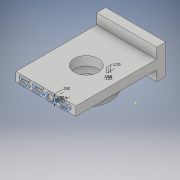
# Autodesk Inventor part: RSL mount
Saved by Autodesk Inventor 2019 (Build 230136000, 136)
## iProperties
Created: 2019-02-11
Part Number: RSL mount
Material: Generic
Document SubType Name: Modeling
Designer: josh
Density: 1 g/cm^3
Appearance: Default
Author: josh
Autodesk Inventor part; units mm, degrees
sketch "Sketch1" plane through (0, 0, 0) normal (0, 0, 1) x (1, 0, 0)
  line L0 (50.8, 31.75) -> (50.8, 57.15)
  line L1 (0, 57.15) -> (0, 31.75)
  line L2 (0, 57.15) -> (0, 48.26)
  line L3 (0, 31.75) -> (0, 40.64)
  line L4 (0, 40.64) -> (50.8, 40.64)
  line L5 (50.8, 48.26) -> (0, 48.26)
  line L6 (0, 40.64) -> (0, 31.75)
  line L7 (0, 31.75) -> (50.8, 31.75)
  line L8 (0, 48.26) -> (0, 57.15)
  line L9 (0, 57.15) -> (50.8, 57.15)
  point P0 (0, 0)
  dimension "d30" = 7.62
  dimension "d33" = 8.89
  dimension "d34" = 8.89
  constraints: 20 end point, 4 perpendicular, 4 point on line, 1 parallel
  measures "d30" distance between parallel lines of L4 L5
  measures "d33" distance of L1.end L3.end
  measures "d34" distance of L1.start L2.end
sketch "Sketch1 outline for Extrusion1" plane through (0, 0, 0) normal (0, 0, 1) x (1, 0, 0)
  line L0 (50.8, 57.15) -> (0, 57.15)
  line L1 (0, 57.15) -> (0, 31.75)
  line L2 (0, 31.75) -> (50.8, 31.75)
  line L3 (50.8, 31.75) -> (50.8, 57.15)
extrude "Extrusion1" add sketch "Sketch1 outline for Extrusion1" along normal blind 7.62
sketch "Sketch1 outline for Extrusion2" plane through (0, 0, 0) normal (0, 0, 1) x (1, 0, 0)
  line L0 (50.8, 48.26) -> (0, 48.26)
  line L1 (50.8, 40.64) -> (50.8, 48.26)
  line L2 (0, 40.64) -> (50.8, 40.64)
  line L3 (0, 48.26) -> (0, 40.64)
extrude "Extrusion2" add sketch "Sketch1 outline for Extrusion2" along normal blind 76.2
sketch "Sketch3" plane through (0, 48.26, 7.62) normal (0, 1, 0) x (1, 0, 0)
  line L0 (0, 0) -> (0, -68.58) projected
  line L1 (0, -34.29) -> (50.8, -34.29)
  line L2 (50.8, 0) -> (50.8, -68.58) projected
  circle A0 centre (25.4, -34.29) radius 10.16
  point P0 (0, 7.62)
  dimension "d8" = 20.32
  constraints: 3 midpoint, 2 end point, 1 centre point
  measures "d8" diameter of A0
sketch "Sketch3 outline for Extrusion3" plane through (0, 48.26, 7.62) normal (0, 1, 0) x (1, 0, 0)
  circle A0 centre (25.4, -34.29) radius 10.16
extrude "Extrusion3" cut sketch "Sketch3 outline for Extrusion3" against normal blind 50.8
sketch "Sketch4" plane through (0, 0, 76.2) normal (0, 0, 1) x (1, 0, 0)
  line L0 (2.114668, 47.727642) -> (47.879129, 47.727642) construction
  line L1 (47.879129, 47.727642) -> (47.879129, 41.3797) construction
  line L2 (47.879129, 41.3797) -> (2.114668, 41.3797) construction
  line L3 (2.114668, 41.3797) -> (2.114668, 47.727642) construction
  spline S0 degree 2 poles (12.464037, 43.444634) (12.464037, 43.004971) (11.757612, 42.254086) (11.125288, 41.977444) knots 0 0 0 1 2 2 2
  spline S1 degree 2 poles (11.125288, 41.977444) (10.478143, 41.700803) (8.566351, 41.3797) (7.375803, 41.3797) knots 0 0 0 1 2 2 2
  spline S2 degree 2 poles (7.375803, 41.3797) (6.279116, 41.3797) (4.159842, 41.572362) (3.384257, 41.725503) knots 0 0 0 1 2 2 2
  line L4 (3.384257, 41.725503) -> (3.384257, 42.590008)
  line L5 (3.384257, 42.590008) -> (3.527518, 42.590008)
  spline S3 degree 2 poles (3.527518, 42.590008) (3.764639, 42.520848) (4.643965, 42.343007) (5.177489, 42.263966) knots 0 0 0 1 2 2 2
  spline S4 degree 2 poles (5.177489, 42.263966) (5.780173, 42.179986) (6.782999, 42.086125) (7.405443, 42.086125) knots 0 0 0 1 2 2 2
  spline S5 degree 2 poles (7.405443, 42.086125) (8.018007, 42.086125) (9.188795, 42.263966) (9.608698, 42.456628) knots 0 0 0 1 2 2 2
  spline S6 degree 2 poles (9.608698, 42.456628) (9.98414, 42.639409) (10.384283, 43.123532) (10.384283, 43.449574) knots 0 0 0 1 2 2 2
  spline S7 degree 2 poles (10.384283, 43.449574) (10.384283, 43.775616) (9.94462, 44.190579) (9.524717, 44.3289) knots 0 0 0 1 2 2 2
  spline S8 degree 2 poles (9.524717, 44.3289) (9.085054, 44.482041) (7.805586, 44.610482) (7.015181, 44.610482) knots 0 0 0 1 2 2 2
  spline S9 degree 2 poles (7.015181, 44.610482) (6.185255, 44.610482) (4.510584, 44.506741) (4.006701, 44.462281) knots 0 0 0 1 2 2 2
  line L6 (4.006701, 44.462281) -> (4.006701, 47.604141)
  line L7 (4.006701, 47.604141) -> (12.370176, 47.604141)
  line L8 (12.370176, 47.604141) -> (12.370176, 46.887837)
  line L9 (12.370176, 46.887837) -> (5.982714, 46.887837)
  line L10 (5.982714, 46.887837) -> (5.982714, 45.262566)
  spline S10 degree 2 poles (5.982714, 45.262566) (6.353216, 45.282326) (7.069521, 45.297146) (7.365923, 45.297146) knots 0 0 0 1 2 2 2
  spline S11 degree 2 poles (7.365923, 45.297146) (8.531771, 45.297146) (10.152101, 45.144005) (10.898046, 44.916764) knots 0 0 0 1 2 2 2
  spline S12 degree 2 poles (10.898046, 44.916764) (11.653871, 44.689522) (12.464037, 43.997918) (12.464037, 43.444634) knots 0 0 0 1 2 2 2
  spline S13 degree 2 poles (23.905152, 43.444634) (23.905152, 43.004971) (23.198727, 42.254086) (22.566403, 41.977444) knots 0 0 0 1 2 2 2
  spline S14 degree 2 poles (22.566403, 41.977444) (21.919259, 41.700803) (20.007466, 41.3797) (18.816918, 41.3797) knots 0 0 0 1 2 2 2
  spline S15 degree 2 poles (18.816918, 41.3797) (17.720231, 41.3797) (15.600957, 41.572362) (14.825372, 41.725503) knots 0 0 0 1 2 2 2
  line L11 (14.825372, 41.725503) -> (14.825372, 42.590008)
  line L12 (14.825372, 42.590008) -> (14.968633, 42.590008)
  spline S16 degree 2 poles (14.968633, 42.590008) (15.205755, 42.520848) (16.08508, 42.343007) (16.618604, 42.263966) knots 0 0 0 1 2 2 2
  spline S17 degree 2 poles (16.618604, 42.263966) (17.221288, 42.179986) (18.224114, 42.086125) (18.846558, 42.086125) knots 0 0 0 1 2 2 2
  spline S18 degree 2 poles (18.846558, 42.086125) (19.459123, 42.086125) (20.62991, 42.263966) (21.049813, 42.456628) knots 0 0 0 1 2 2 2
  spline S19 degree 2 poles (21.049813, 42.456628) (21.425255, 42.639409) (21.825398, 43.123532) (21.825398, 43.449574) knots 0 0 0 1 2 2 2
  spline S20 degree 2 poles (21.825398, 43.449574) (21.825398, 43.775616) (21.385735, 44.190579) (20.965832, 44.3289) knots 0 0 0 1 2 2 2
  spline S21 degree 2 poles (20.965832, 44.3289) (20.52617, 44.482041) (19.246701, 44.610482) (18.456296, 44.610482) knots 0 0 0 1 2 2 2
  spline S22 degree 2 poles (18.456296, 44.610482) (17.62637, 44.610482) (15.951699, 44.506741) (15.447816, 44.462281) knots 0 0 0 1 2 2 2
  line L13 (15.447816, 44.462281) -> (15.447816, 47.604141)
  line L14 (15.447816, 47.604141) -> (23.811291, 47.604141)
  line L15 (23.811291, 47.604141) -> (23.811291, 46.887837)
  line L16 (23.811291, 46.887837) -> (17.423829, 46.887837)
  line L17 (17.423829, 46.887837) -> (17.423829, 45.262566)
  spline S23 degree 2 poles (17.423829, 45.262566) (17.794332, 45.282326) (18.510636, 45.297146) (18.807038, 45.297146) knots 0 0 0 1 2 2 2
  spline S24 degree 2 poles (18.807038, 45.297146) (19.972886, 45.297146) (21.593217, 45.144005) (22.339161, 44.916764) knots 0 0 0 1 2 2 2
  spline S25 degree 2 poles (22.339161, 44.916764) (23.094986, 44.689522) (23.905152, 43.997918) (23.905152, 43.444634) knots 0 0 0 1 2 2 2
  spline S26 degree 2 poles (35.588329, 44.556141) (35.588329, 42.916051) (33.202293, 41.3797) (30.717457, 41.3797) knots 0 0 0 1 2 2 2
  spline S27 degree 2 poles (30.717457, 41.3797) (28.19804, 41.3797) (25.846585, 42.945691) (25.846585, 44.551201) knots 0 0 0 1 2 2 2
  spline S28 degree 2 poles (25.846585, 44.551201) (25.846585, 46.201172) (28.23262, 47.727642) (30.717457, 47.727642) knots 0 0 0 1 2 2 2
  spline S29 degree 2 poles (30.717457, 47.727642) (33.236873, 47.727642) (35.588329, 46.146832) (35.588329, 44.556141) knots 0 0 0 1 2 2 2
  spline S30 degree 2 poles (32.965171, 42.698689) (33.261573, 43.000031) (33.508575, 43.928757) (33.508575, 44.556141) knots 0 0 0 1 2 2 2
  spline S31 degree 2 poles (33.508575, 44.556141) (33.508575, 45.183525) (33.261573, 46.107312) (32.955291, 46.418534) knots 0 0 0 1 2 2 2
  spline S32 degree 2 poles (32.955291, 46.418534) (32.649009, 46.729756) (31.577022, 47.050858) (30.717457, 47.050858) knots 0 0 0 1 2 2 2
  spline S33 degree 2 poles (30.717457, 47.050858) (29.867771, 47.050858) (28.776024, 46.729756) (28.459862, 46.408654) knots 0 0 0 1 2 2 2
  spline S34 degree 2 poles (28.459862, 46.408654) (28.15358, 46.097431) (27.926338, 45.148945) (27.926338, 44.551201) knots 0 0 0 1 2 2 2
  spline S35 degree 2 poles (27.926338, 44.551201) (27.926338, 43.908997) (28.118999, 43.049431) (28.449982, 42.713509) knots 0 0 0 1 2 2 2
  spline S36 degree 2 poles (28.449982, 42.713509) (28.746384, 42.397347) (29.838131, 42.056485) (30.717457, 42.056485) knots 0 0 0 1 2 2 2
  spline S37 degree 2 poles (30.717457, 42.056485) (31.567142, 42.056485) (32.658889, 42.377587) (32.965171, 42.698689) knots 0 0 0 1 2 2 2
  spline S38 degree 2 poles (37.124679, 45.623188) (37.124679, 46.092491) (37.890384, 46.873017) (38.557288, 47.154598) knots 0 0 0 1 2 2 2
  spline S39 degree 2 poles (38.557288, 47.154598) (39.189612, 47.4263) (41.022364, 47.727642) (41.96591, 47.727642) knots 0 0 0 1 2 2 2
  spline S40 degree 2 poles (41.96591, 47.727642) (43.018137, 47.727642) (44.727389, 47.44606) (45.349833, 47.179299) knots 0 0 0 1 2 2 2
  spline S41 degree 2 poles (45.349833, 47.179299) (46.140238, 46.843376) (47.009684, 45.756569) (47.009684, 44.921704) knots 0 0 0 1 2 2 2
  spline S42 degree 2 poles (47.009684, 44.921704) (47.009684, 44.165879) (46.159998, 42.81231) (45.330073, 42.362767) knots 0 0 0 1 2 2 2
  spline S43 degree 2 poles (45.330073, 42.362767) (44.450747, 41.888524) (41.985671, 41.389581) (40.172679, 41.389581) knots 0 0 0 1 2 2 2
  spline S44 degree 2 poles (40.172679, 41.389581) (39.762656, 41.389581) (38.84381, 41.424161) (38.443667, 41.473561) knots 0 0 0 1 2 2 2
  line L18 (38.443667, 41.473561) -> (38.443667, 42.259026)
  line L19 (38.443667, 42.259026) -> (38.547408, 42.259026)
  spline S45 degree 2 poles (38.547408, 42.259026) (38.80429, 42.199746) (39.886157, 42.096005) (40.449321, 42.096005) knots 0 0 0 1 2 2 2
  spline S46 degree 2 poles (40.449321, 42.096005) (42.454974, 42.096005) (44.752089, 43.153172) (44.90523, 44.131299) knots 0 0 0 1 2 2 2
  spline S47 degree 2 poles (44.90523, 44.131299) (44.085184, 43.908997) (42.598235, 43.706456) (41.728789, 43.706456) knots 0 0 0 1 2 2 2
  spline S48 degree 2 poles (41.728789, 43.706456) (40.879103, 43.706456) (39.490954, 43.854657) (38.78453, 44.067078) knots 0 0 0 1 2 2 2
  spline S49 degree 2 poles (38.78453, 44.067078) (37.964484, 44.31902) (37.124679, 45.084725) (37.124679, 45.623188) knots 0 0 0 1 2 2 2
  spline S50 degree 2 poles (44.95463, 45.104485) (44.95463, 45.721989) (44.381586, 46.502514) (43.882643, 46.714936) knots 0 0 0 1 2 2 2
  spline S51 degree 2 poles (43.882643, 46.714936) (43.42816, 46.912537) (42.509314, 47.060738) (41.95603, 47.060738) knots 0 0 0 1 2 2 2
  spline S52 degree 2 poles (41.95603, 47.060738) (40.696322, 47.060738) (39.204432, 46.339493) (39.204432, 45.657769) knots 0 0 0 1 2 2 2
  spline S53 degree 2 poles (39.204432, 45.657769) (39.204432, 45.272446) (39.693496, 44.773503) (40.246779, 44.595662) knots 0 0 0 1 2 2 2
  spline S54 degree 2 poles (40.246779, 44.595662) (40.637042, 44.467221) (41.620108, 44.38324) (42.183272, 44.38324) knots 0 0 0 1 2 2 2
  spline S55 degree 2 poles (42.183272, 44.38324) (42.835356, 44.38324) (44.351946, 44.566021) (44.91511, 44.719162) knots 0 0 0 1 2 2 2
  spline S56 degree 2 poles (44.91511, 44.719162) (44.92499, 44.778443) (44.95463, 44.980984) (44.95463, 45.104485) knots 0 0 0 1 2 2 2
  point P0 (0, 0)
  constraints: 2 other
sketch "Sketch4 outline for Emboss1" plane through (0, 0, 76.2) normal (0, 0, 1) x (1, 0, 0)
  spline S0 degree 2 poles (12.464037, 43.444634) (12.464037, 43.004971) (11.757612, 42.254086) (11.125288, 41.977444) knots 0 0 0 0.5 1 1 1
  spline S1 degree 2 poles (11.125288, 41.977444) (10.478143, 41.700803) (8.566351, 41.3797) (7.375803, 41.3797) knots 0 0 0 0.5 1 1 1
  spline S2 degree 2 poles (7.375803, 41.3797) (6.279116, 41.3797) (4.159842, 41.572362) (3.384257, 41.725503) knots 0 0 0 0.5 1 1 1
  line L0 (3.384257, 41.725503) -> (3.384257, 42.590008)
  line L1 (3.384257, 42.590008) -> (3.527518, 42.590008)
  spline S3 degree 2 poles (3.527518, 42.590008) (3.764639, 42.520848) (4.643965, 42.343007) (5.177489, 42.263966) knots 0 0 0 0.5 1 1 1
  spline S4 degree 2 poles (5.177489, 42.263966) (5.780173, 42.179986) (6.782999, 42.086125) (7.405443, 42.086125) knots 0 0 0 0.5 1 1 1
  spline S5 degree 2 poles (7.405443, 42.086125) (8.018007, 42.086125) (9.188795, 42.263966) (9.608698, 42.456628) knots 0 0 0 0.5 1 1 1
  spline S6 degree 2 poles (9.608698, 42.456628) (9.98414, 42.639409) (10.384283, 43.123532) (10.384283, 43.449574) knots 0 0 0 0.5 1 1 1
  spline S7 degree 2 poles (10.384283, 43.449574) (10.384283, 43.775616) (9.94462, 44.190579) (9.524717, 44.3289) knots 0 0 0 0.5 1 1 1
  spline S8 degree 2 poles (9.524717, 44.3289) (9.085054, 44.482041) (7.805586, 44.610482) (7.015181, 44.610482) knots 0 0 0 0.5 1 1 1
  spline S9 degree 2 poles (7.015181, 44.610482) (6.185255, 44.610482) (4.510584, 44.506741) (4.006701, 44.462281) knots 0 0 0 0.5 1 1 1
  line L2 (4.006701, 44.462281) -> (4.006701, 47.604141)
  line L3 (4.006701, 47.604141) -> (12.370176, 47.604141)
  line L4 (12.370176, 47.604141) -> (12.370176, 46.887837)
  line L5 (12.370176, 46.887837) -> (5.982714, 46.887837)
  line L6 (5.982714, 46.887837) -> (5.982714, 45.262566)
  spline S10 degree 2 poles (5.982714, 45.262566) (6.353216, 45.282326) (7.069521, 45.297146) (7.365923, 45.297146) knots 0 0 0 0.5 1 1 1
  spline S11 degree 2 poles (7.365923, 45.297146) (8.531771, 45.297146) (10.152101, 45.144005) (10.898046, 44.916764) knots 0 0 0 0.5 1 1 1
  spline S12 degree 2 poles (10.898046, 44.916764) (11.653871, 44.689522) (12.464037, 43.997918) (12.464037, 43.444634) knots 0 0 0 0.5 1 1 1
  spline S13 degree 2 poles (23.905152, 43.444634) (23.905152, 43.004971) (23.198727, 42.254086) (22.566403, 41.977444) knots 0 0 0 0.5 1 1 1
  spline S14 degree 2 poles (22.566403, 41.977444) (21.919259, 41.700803) (20.007466, 41.3797) (18.816918, 41.3797) knots 0 0 0 0.5 1 1 1
  spline S15 degree 2 poles (18.816918, 41.3797) (17.720231, 41.3797) (15.600957, 41.572362) (14.825372, 41.725503) knots 0 0 0 0.5 1 1 1
  line L7 (14.825372, 41.725503) -> (14.825372, 42.590008)
  line L8 (14.825372, 42.590008) -> (14.968633, 42.590008)
  spline S16 degree 2 poles (14.968633, 42.590008) (15.205755, 42.520848) (16.08508, 42.343007) (16.618604, 42.263966) knots 0 0 0 0.5 1 1 1
  spline S17 degree 2 poles (16.618604, 42.263966) (17.221288, 42.179986) (18.224114, 42.086125) (18.846558, 42.086125) knots 0 0 0 0.5 1 1 1
  spline S18 degree 2 poles (18.846558, 42.086125) (19.459123, 42.086125) (20.62991, 42.263966) (21.049813, 42.456628) knots 0 0 0 0.5 1 1 1
  spline S19 degree 2 poles (21.049813, 42.456628) (21.425255, 42.639409) (21.825398, 43.123532) (21.825398, 43.449574) knots 0 0 0 0.5 1 1 1
  spline S20 degree 2 poles (21.825398, 43.449574) (21.825398, 43.775616) (21.385735, 44.190579) (20.965832, 44.3289) knots 0 0 0 0.5 1 1 1
  spline S21 degree 2 poles (20.965832, 44.3289) (20.52617, 44.482041) (19.246701, 44.610482) (18.456296, 44.610482) knots 0 0 0 0.5 1 1 1
  spline S22 degree 2 poles (18.456296, 44.610482) (17.62637, 44.610482) (15.951699, 44.506741) (15.447816, 44.462281) knots 0 0 0 0.5 1 1 1
  line L9 (15.447816, 44.462281) -> (15.447816, 47.604141)
  line L10 (15.447816, 47.604141) -> (23.811291, 47.604141)
  line L11 (23.811291, 47.604141) -> (23.811291, 46.887837)
  line L12 (23.811291, 46.887837) -> (17.423829, 46.887837)
  line L13 (17.423829, 46.887837) -> (17.423829, 45.262566)
  spline S23 degree 2 poles (17.423829, 45.262566) (17.794332, 45.282326) (18.510636, 45.297146) (18.807038, 45.297146) knots 0 0 0 0.5 1 1 1
  spline S24 degree 2 poles (18.807038, 45.297146) (19.972886, 45.297146) (21.593217, 45.144005) (22.339161, 44.916764) knots 0 0 0 0.5 1 1 1
  spline S25 degree 2 poles (22.339161, 44.916764) (23.094986, 44.689522) (23.905152, 43.997918) (23.905152, 43.444634) knots 0 0 0 0.5 1 1 1
  spline S26 degree 2 poles (35.588329, 44.556141) (35.588329, 42.916051) (33.202293, 41.3797) (30.717457, 41.3797) knots 0 0 0 0.5 1 1 1
  spline S27 degree 2 poles (30.717457, 47.727642) (33.236873, 47.727642) (35.588329, 46.146832) (35.588329, 44.556141) knots 0 0 0 0.5 1 1 1
  spline S28 degree 2 poles (30.717457, 41.3797) (28.19804, 41.3797) (25.846585, 42.945691) (25.846585, 44.551201) knots 0 0 0 0.5 1 1 1
  spline S29 degree 2 poles (25.846585, 44.551201) (25.846585, 46.201172) (28.23262, 47.727642) (30.717457, 47.727642) knots 0 0 0 0.5 1 1 1
  spline S30 degree 2 poles (30.717457, 42.056485) (31.567142, 42.056485) (32.658889, 42.377587) (32.965171, 42.698689) knots 0 0 0 0.5 1 1 1
  spline S31 degree 2 poles (32.965171, 42.698689) (33.261573, 43.000031) (33.508575, 43.928757) (33.508575, 44.556141) knots 0 0 0 0.5 1 1 1
  spline S32 degree 2 poles (33.508575, 44.556141) (33.508575, 45.183525) (33.261573, 46.107312) (32.955291, 46.418534) knots 0 0 0 0.5 1 1 1
  spline S33 degree 2 poles (32.955291, 46.418534) (32.649009, 46.729756) (31.577022, 47.050858) (30.717457, 47.050858) knots 0 0 0 0.5 1 1 1
  spline S34 degree 2 poles (30.717457, 47.050858) (29.867771, 47.050858) (28.776024, 46.729756) (28.459862, 46.408654) knots 0 0 0 0.5 1 1 1
  spline S35 degree 2 poles (28.459862, 46.408654) (28.15358, 46.097431) (27.926338, 45.148945) (27.926338, 44.551201) knots 0 0 0 0.5 1 1 1
  spline S36 degree 2 poles (27.926338, 44.551201) (27.926338, 43.908997) (28.118999, 43.049431) (28.449982, 42.713509) knots 0 0 0 0.5 1 1 1
  spline S37 degree 2 poles (28.449982, 42.713509) (28.746384, 42.397347) (29.838131, 42.056485) (30.717457, 42.056485) knots 0 0 0 0.5 1 1 1
  spline S38 degree 2 poles (37.124679, 45.623188) (37.124679, 46.092491) (37.890384, 46.873017) (38.557288, 47.154598) knots 0 0 0 0.5 1 1 1
  spline S39 degree 2 poles (38.78453, 44.067078) (37.964484, 44.31902) (37.124679, 45.084725) (37.124679, 45.623188) knots 0 0 0 0.5 1 1 1
  spline S40 degree 2 poles (38.557288, 47.154598) (39.189612, 47.4263) (41.022364, 47.727642) (41.96591, 47.727642) knots 0 0 0 0.5 1 1 1
  spline S41 degree 2 poles (41.728789, 43.706456) (40.879103, 43.706456) (39.490954, 43.854657) (38.78453, 44.067078) knots 0 0 0 0.5 1 1 1
  spline S42 degree 2 poles (41.96591, 47.727642) (43.018137, 47.727642) (44.727389, 47.44606) (45.349833, 47.179299) knots 0 0 0 0.5 1 1 1
  spline S43 degree 2 poles (44.90523, 44.131299) (44.085184, 43.908997) (42.598235, 43.706456) (41.728789, 43.706456) knots 0 0 0 0.5 1 1 1
  spline S44 degree 2 poles (45.349833, 47.179299) (46.140238, 46.843376) (47.009684, 45.756569) (47.009684, 44.921704) knots 0 0 0 0.5 1 1 1
  spline S45 degree 2 poles (40.449321, 42.096005) (42.454974, 42.096005) (44.752089, 43.153172) (44.90523, 44.131299) knots 0 0 0 0.5 1 1 1
  spline S46 degree 2 poles (47.009684, 44.921704) (47.009684, 44.165879) (46.159998, 42.81231) (45.330073, 42.362767) knots 0 0 0 0.5 1 1 1
  spline S47 degree 2 poles (38.547408, 42.259026) (38.80429, 42.199746) (39.886157, 42.096005) (40.449321, 42.096005) knots 0 0 0 0.5 1 1 1
  spline S48 degree 2 poles (45.330073, 42.362767) (44.450747, 41.888524) (41.985671, 41.389581) (40.172679, 41.389581) knots 0 0 0 0.5 1 1 1
  line L14 (38.443667, 42.259026) -> (38.547408, 42.259026)
  spline S49 degree 2 poles (40.172679, 41.389581) (39.762656, 41.389581) (38.84381, 41.424161) (38.443667, 41.473561) knots 0 0 0 0.5 1 1 1
  line L15 (38.443667, 41.473561) -> (38.443667, 42.259026)
  spline S50 degree 2 poles (44.91511, 44.719162) (44.92499, 44.778443) (44.95463, 44.980984) (44.95463, 45.104485) knots 0 0 0 0.5 1 1 1
  spline S51 degree 2 poles (44.95463, 45.104485) (44.95463, 45.721989) (44.381586, 46.502514) (43.882643, 46.714936) knots 0 0 0 0.5 1 1 1
  spline S52 degree 2 poles (43.882643, 46.714936) (43.42816, 46.912537) (42.509314, 47.060738) (41.95603, 47.060738) knots 0 0 0 0.5 1 1 1
  spline S53 degree 2 poles (41.95603, 47.060738) (40.696322, 47.060738) (39.204432, 46.339493) (39.204432, 45.657769) knots 0 0 0 0.5 1 1 1
  spline S54 degree 2 poles (39.204432, 45.657769) (39.204432, 45.272446) (39.693496, 44.773503) (40.246779, 44.595662) knots 0 0 0 0.5 1 1 1
  spline S55 degree 2 poles (40.246779, 44.595662) (40.637042, 44.467221) (41.620108, 44.38324) (42.183272, 44.38324) knots 0 0 0 0.5 1 1 1
  spline S56 degree 2 poles (42.183272, 44.38324) (42.835356, 44.38324) (44.351946, 44.566021) (44.91511, 44.719162) knots 0 0 0 0.5 1 1 1
emboss "Emboss1" sketch "Sketch4 outline for Emboss1" operation add depth 1.27 direction (0, 0, -1)
ref_plane "Work Plane1" through (25.4, 0, 0) normal (1, 0, 0) x (0, 1, 0)
sketch "Sketch5" plane through (25.4, 0, 0) normal (1, 0, 0) x (0, 1, 0)
  line L0 (40.64, 56.014) -> (32.131, 56.014)
  line L1 (40.64, 27.806) -> (32.131, 27.806)
  line L2 (40.64, 56.014) -> (40.64, 62.364)
  line L3 (32.131, 62.364) -> (32.131, 56.014)
  line L4 (32.131, 27.806) -> (32.131, 21.456)
  line L5 (32.131, 62.364) -> (36.3855, 62.364)
  line L6 (36.3855, 62.364) -> (36.3855, 61.094)
  line L7 (36.3855, 61.094) -> (33.8455, 61.094)
  line L8 (33.8455, 61.094) -> (33.8455, 59.189)
  line L9 (33.8455, 59.189) -> (38.1635, 59.189)
  line L10 (38.1635, 59.189) -> (38.1635, 62.364)
  line L11 (38.1635, 21.456) -> (38.1635, 24.631)
  line L12 (38.1635, 24.631) -> (33.8455, 24.631)
  line L13 (33.8455, 24.631) -> (33.8455, 22.726)
  line L14 (33.8455, 22.726) -> (36.3855, 22.726)
  line L15 (36.3855, 22.726) -> (36.3855, 21.456)
  line L16 (40.64, 41.91) -> (13.361908, 41.91)
  line L17 (40.64, 21.456) -> (38.1635, 21.456)
  line L18 (36.3855, 21.456) -> (32.131, 21.456)
  line L19 (40.64, 62.364) -> (38.1635, 62.364)
  line L20 (36.3855, 62.364) -> (32.131, 62.364)
  line L21 (40.64, 21.456) -> (40.64, 27.806)
  point P0 (0, 0)
  dimension "d15" = 8.509
  dimension "d18" = 6.35
  dimension "d19" = 1.27
  dimension "d20" = 2.54
  dimension "d21" = 4.318
  dimension "d22" = 3.175
  dimension "d23" = 4.318
  dimension "d25" = 1.27
  constraints: 44 end point, 8 perpendicular, 3 vertical, 2 horizontal, 1 collinear, 1 parallel
  measures "d15" distance of L0.start L0.end
  measures "d18" distance of L0.start L2.end
  measures "d19" distance of L5.end L6.end
  measures "d20" distance of L6.end L7.end
  measures "d21" distance of L8.end L9.end
  measures "d22" distance of L11.start L11.end
  measures "d23" distance of L11.end L12.end
  measures "d25" distance of L14.end L15.end
sketch "Sketch5 outline for Revolution1" plane through (25.4, 0, 0) normal (1, 0, 0) x (0, 1, 0)
  line L0 (40.64, 21.456) -> (40.64, 27.806)
  line L1 (38.1635, 21.456) -> (40.64, 21.456)
  line L2 (38.1635, 24.631) -> (38.1635, 21.456)
  line L3 (33.8455, 24.631) -> (38.1635, 24.631)
  line L4 (33.8455, 22.726) -> (33.8455, 24.631)
  line L5 (36.3855, 22.726) -> (33.8455, 22.726)
  line L6 (36.3855, 21.456) -> (36.3855, 22.726)
  line L7 (32.131, 21.456) -> (36.3855, 21.456)
  line L8 (32.131, 27.806) -> (32.131, 21.456)
  line L9 (40.64, 27.806) -> (32.131, 27.806)
  line L10 (32.131, 56.014) -> (40.64, 56.014)
  line L11 (32.131, 62.364) -> (32.131, 56.014)
  line L12 (36.3855, 62.364) -> (32.131, 62.364)
  line L13 (36.3855, 61.094) -> (36.3855, 62.364)
  line L14 (33.8455, 61.094) -> (36.3855, 61.094)
  line L15 (33.8455, 59.189) -> (33.8455, 61.094)
  line L16 (38.1635, 59.189) -> (33.8455, 59.189)
  line L17 (38.1635, 62.364) -> (38.1635, 59.189)
  line L18 (40.64, 62.364) -> (38.1635, 62.364)
  line L19 (40.64, 56.014) -> (40.64, 62.364)
revolve "Revolution1" add sketch "Sketch5 outline for Revolution1" angle 15 about axis through (25.4, 40.64, 41.91) along (0, -1, 0)
ref_plane "Work Plane2" through (20.106115, 38.1635, 61.667047) normal (-0.9659258, 0, -0.258819) x (0, -1, 0)
sketch "Sketch6" plane through (20.106115, 38.1635, 61.667047) normal (-0.9659258, 0, -0.258819) x (0, -1, 0)
  line L0 (-2.4765, -6.35) -> (-2.4765, 0)
  line L1 (-2.4765, -6.35) -> (6.0325, -6.35)
  line L2 (6.0325, -6.35) -> (6.0325, 0)
  line L3 (6.0325, 0) -> (1.778, 0)
  line L4 (1.778, 0) -> (1.778, -1.27)
  line L5 (1.778, -1.27) -> (4.318, -1.27)
  line L6 (4.318, -1.27) -> (4.318, -3.175)
  line L7 (4.318, -3.175) -> (0, -3.175)
  line L8 (0, -3.175) -> (0, 0)
  line L9 (0, 0) -> (-2.4765, 0)
  line L10 (1.778, 0) -> (1.778, -1.27)
  line L11 (1.778, -1.27) -> (1.778, -3.175)
  line L12 (1.778, 0) -> (1.778, -1.27)
  line L13 (-2.4765, -6.35) -> (6.0325, -6.35)
  line L14 (6.0325, -6.35) -> (6.0325, 0)
  line L15 (-2.4765, 0) -> (-2.4765, -6.35)
  line L16 (6.0325, 0) -> (1.778, 0)
  line L17 (0, 0) -> (-2.4765, 0)
  line L18 (0, -3.175) -> (0, 0)
  line L19 (1.778, -3.175) -> (0, -3.175)
  line L20 (0, -3.175) -> (0, 0)
  line L21 (-2.4765, -34.558) -> (6.0325, -34.558)
  line L22 (6.0325, -34.558) -> (6.0325, -40.908)
  line L23 (6.0325, -40.908) -> (1.778, -40.908)
  line L24 (1.778, -40.908) -> (1.778, -39.638)
  line L25 (1.778, -39.638) -> (4.318, -39.638)
  line L26 (4.318, -39.638) -> (4.318, -37.733)
  line L27 (4.318, -37.733) -> (0, -37.733)
  line L28 (0, -37.733) -> (0, -40.908)
  line L29 (0, -40.908) -> (-2.4765, -40.908)
  line L30 (-2.4765, -34.558) -> (-2.4765, -40.908)
  line L31 (1.778, -40.908) -> (1.778, -37.733)
  line L32 (4.318, -37.733) -> (0, -37.733)
  line L33 (1.778, -37.733) -> (0, -37.733)
  line L34 (0, -37.733) -> (0, -40.908)
  line L35 (-2.4765, -34.558) -> (6.0325, -34.558)
  line L36 (6.0325, -34.558) -> (6.0325, -40.908)
  line L37 (-2.4765, -40.908) -> (-2.4765, -34.558)
  line L38 (6.0325, -40.908) -> (1.778, -40.908)
  line L39 (0, -40.908) -> (-2.4765, -40.908)
  line L40 (-2.4765, 0) -> (-2.4765, -40.908)
  line L41 (-2.4765, -47.001593) -> (-2.4765, 19.2416)
  line L42 (-2.4765, -20.454) -> (9.138689, -20.454)
  point P0 (38.1635, -54.361948)
  constraints: 39 end point, 6 parallel, 6 perpendicular, 4 horizontal, 2 collinear, 2 point on line, 1 midpoint, 1 vertical
sketch "Sketch6 outline for Revolution2" plane through (20.106115, 38.1635, 61.667047) normal (-0.9659258, 0, -0.258819) x (0, -1, 0)
  line L0 (1.778, -3.175) -> (0, -3.175)
  line L1 (0, -3.175) -> (0, 0)
  line L2 (0, 0) -> (-2.4765, 0)
  line L3 (-2.4765, 0) -> (-2.4765, -6.35)
  line L4 (-2.4765, -6.35) -> (6.0325, -6.35)
  line L5 (6.0325, -6.35) -> (6.0325, 0)
  line L6 (6.0325, 0) -> (1.778, 0)
  line L7 (1.778, 0) -> (1.778, -3.175)
  line L8 (0, -37.733) -> (1.778, -37.733)
  line L9 (0, -40.908) -> (0, -37.733)
  line L10 (-2.4765, -40.908) -> (0, -40.908)
  line L11 (-2.4765, -34.558) -> (-2.4765, -40.908)
  line L12 (6.0325, -34.558) -> (-2.4765, -34.558)
  line L13 (6.0325, -40.908) -> (6.0325, -34.558)
  line L14 (1.778, -40.908) -> (6.0325, -40.908)
  line L15 (1.778, -37.733) -> (1.778, -40.908)
revolve "Revolution2" add sketch "Sketch6 outline for Revolution2" angle 20 about axis through (25.4, 40.64, 41.91) along (0, -1, 0)
ref_plane "Work Plane3" through (25.4, 36.3855, 62.364) normal (-1, 0, 0) x (0, -1, 0)
sketch "Sketch7" plane through (25.4, 36.3855, 62.364) normal (-1, 0, 0) x (0, -1, 0)
  line L0 (-4.2545, 0) -> (-4.2545, -6.35) projected
  line L1 (-4.2545, 0) -> (-1.778, 0) projected
  line L2 (0, 0) -> (4.2545, 0) projected
  line L3 (4.2545, 0) -> (4.2545, -6.35) projected
  line L4 (4.2545, -6.35) -> (-4.2545, -6.35) projected
  line L5 (-4.2545, -34.558) -> (4.2545, -34.558) projected
  line L6 (-4.2545, -40.908) -> (-4.2545, -34.558) projected
  line L7 (-1.778, -40.908) -> (-4.2545, -40.908) projected
  line L8 (4.2545, -40.908) -> (0, -40.908) projected
  line L9 (4.2545, -34.558) -> (4.2545, -40.908) projected
  line L10 (-4.2545, 0) -> (4.2545, 0)
  line L11 (4.2545, 0) -> (4.2545, -6.35)
  line L12 (4.2545, -6.35) -> (-4.2545, -6.35)
  line L13 (-4.2545, -6.35) -> (-4.2545, 0)
  line L14 (-4.2545, -40.908) -> (4.2545, -40.908)
  line L15 (4.2545, -40.908) -> (4.2545, -34.558)
  line L16 (4.2545, -34.558) -> (-4.2545, -34.558)
  line L17 (-4.2545, -34.558) -> (-4.2545, -40.908)
  line L18 (-4.2545, -40.908) -> (-4.2545, 0)
  line L19 (-4.2545, -20.454) -> (4.2545, -20.454)
  point P0 (36.3855, -62.364)
  point P1 (-1.778, -3.175)
  constraints: 20 end point, 4 parallel, 3 horizontal, 2 perpendicular, 1 midpoint, 1 vertical
sketch "Sketch7 outline for Revolution3" plane through (25.4, 36.3855, 62.364) normal (-1, 0, 0) x (0, -1, 0)
  line L0 (4.2545, 0) -> (-4.2545, 0)
  line L1 (4.2545, -6.35) -> (4.2545, 0)
  line L2 (-4.2545, -6.35) -> (4.2545, -6.35)
  line L3 (-4.2545, 0) -> (-4.2545, -6.35)
  line L4 (-4.2545, -34.558) -> (-4.2545, -40.908)
  line L5 (4.2545, -34.558) -> (-4.2545, -34.558)
  line L6 (4.2545, -40.908) -> (4.2545, -34.558)
  line L7 (-4.2545, -40.908) -> (4.2545, -40.908)
revolve "Revolution3" add sketch "Sketch7 outline for Revolution3" angle 130 about axis through (25.4, 40.64, 41.91) along (0, 1, 0)
ref_plane "Work Plane4" through (13.668068, 36.3855, 58.664936) normal (-0.819152, 0, -0.5735764) x (0, -1, 0)
sketch "Sketch8" plane through (13.668068, 36.3855, 58.664936) normal (-0.819152, 0, -0.5735764) x (0, -1, 0)
  line L0 (0, -3.175) -> (-1.778, -3.175)
  line L1 (-1.778, -3.175) -> (-1.778, 0)
  line L2 (-1.778, 0) -> (-4.2545, 0)
  line L3 (-4.2545, -6.35) -> (-4.2545, 0)
  line L4 (-4.2545, -6.35) -> (4.2545, -6.35)
  line L5 (4.2545, -6.35) -> (4.2545, 0)
  line L6 (4.2545, 0) -> (0, 0)
  line L7 (0, 0) -> (0, -3.175)
  line L8 (0, -40.908) -> (0, -37.733)
  line L9 (0, -37.733) -> (-1.778, -37.733)
  line L10 (-1.778, -37.733) -> (-1.778, -40.908)
  line L11 (-1.778, -40.908) -> (-4.2545, -40.908)
  line L12 (-4.2545, -34.558) -> (-4.2545, -40.908)
  line L13 (-4.2545, -34.558) -> (4.2545, -34.558)
  line L14 (4.2545, -34.558) -> (4.2545, -40.908)
  line L15 (4.2545, -40.908) -> (0, -40.908)
  line L16 (-1.778, -37.733) -> (-1.778, -34.608128)
  line L17 (-1.778, -37.733) -> (4.2545, -37.733)
  line L18 (4.2545, -34.558) -> (-4.2545, -34.558)
  line L19 (4.2545, -40.908) -> (0, -40.908)
  line L20 (-4.2545, -34.558) -> (-4.2545, -40.908)
  line L21 (-4.2545, -40.908) -> (-1.778, -40.908)
  line L22 (-1.778, -37.733) -> (-1.778, -40.908)
  line L23 (-4.2545, -6.35) -> (4.2545, -6.35)
  line L24 (4.2545, -6.35) -> (-4.2545, -6.35)
  line L25 (-4.2545, -6.35) -> (-4.2545, 0)
  line L26 (-1.778, 0) -> (-1.778, -3.175)
  line L27 (0, -3.175) -> (-1.778, -3.175)
  line L28 (-1.778, -3.175) -> (4.2545, -3.175)
  line L29 (4.2545, -6.35) -> (4.2545, 0)
  line L30 (4.2545, -3.175) -> (4.2545, -6.35)
  line L31 (-1.778, -40.908) -> (-4.2545, -40.908)
  line L32 (-4.2545, -40.908) -> (-4.2545, 0)
  line L33 (-4.2545, -20.454) -> (21.138744, -20.454)
  point P0 (36.3855, -40.215821)
  constraints: 22 end point, 3 collinear, 3 midpoint, 3 perpendicular, 1 horizontal, 1 parallel
sketch "Sketch8 outline for Revolution4" plane through (13.668068, 36.3855, 58.664936) normal (-0.819152, 0, -0.5735764) x (0, -1, 0)
  line L0 (4.2545, -3.175) -> (-1.778, -3.175)
  line L1 (4.2545, -6.35) -> (4.2545, -3.175)
  line L2 (-4.2545, -6.35) -> (4.2545, -6.35)
  line L3 (-4.2545, 0) -> (-4.2545, -6.35)
  line L4 (-1.778, 0) -> (-4.2545, 0)
  line L5 (-1.778, -3.175) -> (-1.778, 0)
  line L6 (-4.2545, -34.558) -> (-4.2545, -40.908)
  line L7 (4.2545, -34.558) -> (-4.2545, -34.558)
  line L8 (4.2545, -37.733) -> (4.2545, -34.558)
  line L9 (-1.778, -37.733) -> (4.2545, -37.733)
  line L10 (-1.778, -40.908) -> (-1.778, -37.733)
  line L11 (-4.2545, -40.908) -> (-1.778, -40.908)
revolve "Revolution4" add sketch "Sketch8 outline for Revolution4" angle 15 about axis through (25.4, 40.64, 41.91) along (0, -1, 0)
body "Solid1"
